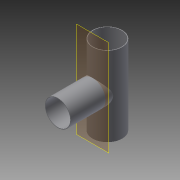
# Autodesk Inventor part: 51mm nipple
Saved by Autodesk Inventor 2015 (Build 190159000, 159)
## iProperties
Created: 2014-05-19
Part Number: 51mm nipple
Material: Generic
Document SubType Name: Modeling
Designer: jad211
Density: 1 g/cm^3
Appearance: Default
Author: jad211
Autodesk Inventor part; units mm, degrees
ref_plane "YZ Plane" through (0, 0, 0) normal (1, 0, 0) x (0, 1, 0)
ref_plane "XZ Plane" through (0, 0, 0) normal (0, 1, 0) x (-1, 0, 0)
sketch "Sketch1" plane through (0, 0, 0) normal (0, 1, 0) x (-1, 0, 0)
  circle A0 centre (0, 0) radius 25.5
  circle A1 centre (0, 0) radius 24.5
  dimension "d0" = 51
  dimension "d1" = 49
  constraints: 2 centre point, 2 coincident
  measures "d0" diameter of A0
  measures "d1" diameter of A1
extrude "Extrusion1" add sketch "Sketch1" along normal blind 136.878
ref_plane "Work Plane1" through (0, 0, 25.5) normal (0, 0, 1) x (1, 0, 0)
sketch "Sketch2" plane through (0, 0, 25.5) normal (0, 0, 1) x (1, 0, 0)
  line L0 (0, 0) -> (28.9243, 0) construction
  line L1 (-25.5, 0) -> (25.5, 0) projected
  circle A0 centre (0, 68.439) radius 21.35
  line L2 (-24.5, 136.878) -> (24.5, 136.878) projected
  dimension "d4" = 42.7
  dimension "d5" = 68.439
  dimension "d18" = 68.439
  constraints: 2 end point, 1 centre point, 1 collinear
  measures "d4" diameter of A0
  measures "d5" distance from line of L0 A0.centre
  measures "d18" distance from line of L2 A0.centre
extrude "Extrusion2" cut sketch "Sketch2" against normal blind 25.4
sketch "Sketch3" plane through (0, 0, 25.5) normal (0, 0, 1) x (1, 0, 0)
  circle A0 centre (0, 68.439) radius 22.35
  line L0 (0, 0) -> (18.5152, 0) construction
  line L1 (24.5, 0) -> (-24.5, 0) projected
  circle A1 centre (0, 68.439) radius 21.35
  dimension "d8" = 68.439
  dimension "d9" = 44.7
  dimension "d10" = 42.7
  constraints: 2 centre point, 2 end point, 1 coincident, 1 point on line
  measures "d8" distance from line of L0 A0.centre
  measures "d9" diameter of A0
  measures "d10" diameter of A1
extrude "Extrusion3" add sketch "Sketch3" along normal blind 60
sketch "Sketch4" plane through (0, 0, 25.5) normal (0, 0, 1) x (1, 0, 0)
  line L0 (0, 0) -> (23.949, 0) construction
  line L1 (24.5, 0) -> (-24.5, 0) projected
  circle A0 centre (0, 68.439) radius 22.35
  circle A1 centre (0, 68.439) radius 21.35
  dimension "d13" = 68.439
  dimension "d14" = 44.7
  dimension "d15" = 42.7
  constraints: 2 centre point, 2 end point, 1 coincident, 1 point on line
  measures "d13" distance from line of L0 A0.centre
  measures "d14" diameter of A0
  measures "d15" diameter of A1
extrude "Extrusion4" add sketch "Sketch4" against normal up to next
equation "\"d5\" = d18"
equation "\"d8\" = d5"
equation "\"d10\" = d4"
equation "\"d13\" = d5"
equation "\"d15\" = d4"
body "Solid1"
